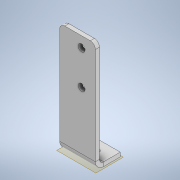
# Autodesk Inventor part: short_bracket_folded
Saved by Autodesk Inventor 2020 (Build 240168000, 168)
## iProperties
Created: 2020-08-23
Part Number: short_bracket_folded
Material: Generic
Document SubType Name: Sheet Metal
Designer: s4393944
Density: 1 g/cm^3
Appearance: Default
Sheet Metal Rule: Default_mm
Flat Pattern Width: 2.6 cm
Flat Pattern Length: 9.358 cm
Flat Pattern Area: 24.3308 cm^2
Sheet Metal Width: 26.000 mm
Sheet Metal Length: 93.580 mm
Sheet Metal Area: 2433.080 mm^2
Author: s4393944
Autodesk Inventor part; units mm, degrees
ref_plane "YZ Plane" through (0, 0, 0) normal (1, 0, 0) x (0, 1, 0)
ref_plane "XY Plane" through (0, 0, 0) normal (0, 0, 1) x (1, 0, 0)
sketch "Sketch2" plane through (0, 0, 0) normal (0, 1, 0) x (-1, 0, 0)
  line L0 (13, 0) -> (13, -15.58)
  line L1 (13, -15.58) -> (-13, -15.58)
  line L2 (-13, -15.58) -> (-13, 0)
  line L3 (13, 0) -> (13, 78)
  line L4 (13, 78) -> (-13, 78)
  line L5 (-13, 78) -> (-13, 0)
  point P0 (0, 0)
extrude "Plate1" add sketch "Sketch2" along normal blind 3
sketch "Sketch3" plane through (0, 3, 0) normal (0, 1, 0) x (1, 0, 0)
  line L0 (-13, -78) -> (-13, 15.58) projected
  line L1 (-13, 0) -> (13, 0)
  line L2 (13, 15.58) -> (13, -78) projected
  point P0 (0, 0)
  constraints: 2 end point, 2 point on line, 1 horizontal
fold "Fold1" angle 90 bend radius 3 thickness 3 k factor 0.44 line from (-13, 3, 0) to (13, 3, 0) line at bend centre moving side (0, 0, 1) folds toward (0, 1, 0)
sketch "Sketch5" plane through (0, 3, 0) normal (0, 1, 0) x (1, 0, 0)
  circle A0 centre (3, 7.3929) radius 2.55
  line L0 (-13, 3.3929) -> (13, 3.3929) projected
  line L1 (13, 15.58) -> (13, 3.3929) projected
  line L2 (-13, 15.58) -> (13, 15.58) projected
  point P0 (0, 0)
  point P1 (-13, 0.3929)
  dimension "d34" = 5.1
  dimension "d35" = 4
  dimension "d36" = 10
  dimension "d57" = 15.1871
  constraints: 1 centre point
  measures "d34" diameter of A0
  measures "d35" distance from line of L0 A0.centre
  measures "d36" distance from line of L1 A0.centre
  measures "d57" distance from line of point (-13, 0.393) L2
hole "Hole2" at (3, 3, -7.3929) direction (0, -1, 0) diameter 5.1 end through all
sketch "Sketch6" plane through (13, 80.6071, -0.3929) normal (0, 0, -1) x (-1, 0, 0)
  circle A0 centre (10, -32.6071) radius 2.55
  circle A1 centre (10, -7.6071) radius 2.55
  line L0 (26, -77.6071) -> (0, -77.6071) projected
  line L1 (0, -74.6071) -> (0, 0) projected
  point P0 (13, -80.6071)
  dimension "d44" = 5.1
  dimension "d45" = 5.1
  dimension "d46" = 45
  dimension "d47" = 70
  dimension "d48" = 10
  dimension "d49" = 10
  constraints: 2 centre point
  measures "d44" diameter of A0
  measures "d45" diameter of A1
  measures "d46" distance from line of L0 A0.centre
  measures "d47" distance from line of L0 A1.centre
  measures "d48" distance from line of L1 A0.centre
  measures "d49" distance from line of L1 A1.centre
hole "Hole3" at (3, 48, -0.3929) at (3, 73, -0.3929) direction (0, 0, 1) diameter 5.1 end through all
fillet "Corner Round1" radius 3.7 2 edges at (-13, 80.6071, 1.1071) (13, 80.6071, 1.1071)
equation "\"d6\" = Thickness"
equation "\"d9\" = BendReliefWidth"
equation "\"d10\" = BendReliefDepth"
equation "\"d11\" = MinimumRemnant"
equation "\"d12\" = TransitionRadius"
equation "\"d14\" = BendRadius"
equation "\"BendRadius\" = Thickness"
equation "\"BendReliefWidth\" = Thickness"
equation "\"BendReliefDepth\" = 0.5 * Thickness"
equation "\"CornerReliefSize\" = 4 * Thickness"
equation "\"MinimumRemnant\" = 2 * Thickness"
equation "\"TransitionRadius\" = BendRadius"
equation "\"JacobiRadiusSize\" = BendRadius"
equation "\"GapSize\" = Thickness"
equation "\"Thickness\" = 3"
body "Solid1"
